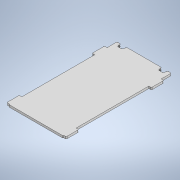
# Autodesk Inventor part: back_wall
Saved by Autodesk Inventor 2020 (Build 240168000, 168)
## iProperties
Created: 2019-06-12
Part Number: back_wall
Material: Generic
Document SubType Name: Modeling
Designer: Dammy
Density: 1 g/cm^3
Appearance: Default
Author: Dammy
Autodesk Inventor part; units mm, degrees
ref_plane "YZ Plane" through (0, 0, 0) normal (1, 0, 0) x (0, 1, 0)
ref_plane "XZ Plane" through (0, 0, 0) normal (0, 1, 0) x (-1, 0, 0)
ref_plane "XY Plane" through (0, 0, 0) normal (0, 0, 1) x (1, 0, 0)
sketch "Sketch1" plane through (0, 0, 0) normal (0, 1, 0) x (-1, 0, 0)
  line L0 (-2, -229.675) -> (-6, -229.675)
  line L1 (-6, -200.675) -> (-2, -200.675)
  line L2 (0, -202.675) -> (0, -227.675)
  line L3 (-6, -30.675) -> (-2, -30.675)
  line L4 (0, -28.675) -> (0, -3.675)
  line L5 (-2, -1.675) -> (-6, -1.675)
  arc A0 (0, -3.675) -> (-2, -1.675) centre (-2, -3.675) ccw
  arc A1 (-2, -30.675) -> (0, -28.675) centre (-2, -28.675) ccw
  arc A2 (0, -202.675) -> (-2, -200.675) centre (-2, -202.675) ccw
  arc A3 (-2, -229.675) -> (0, -227.675) centre (-2, -227.675) ccw
  line L6 (-136.5, -229.675) -> (-132.5, -229.675)
  line L7 (-132.5, -200.675) -> (-136.5, -200.675)
  line L8 (-138.5, -202.675) -> (-138.5, -227.675)
  line L9 (-136.5, -30.675) -> (-132.5, -30.675)
  line L10 (-132.5, -1.675) -> (-136.5, -1.675)
  line L11 (-138.5, -3.675) -> (-138.5, -28.675)
  arc A4 (-136.5, -1.675) -> (-138.5, -3.675) centre (-136.5, -3.675) ccw
  arc A5 (-138.5, -28.675) -> (-136.5, -30.675) centre (-136.5, -28.675) ccw
  arc A6 (-136.5, -200.675) -> (-138.5, -202.675) centre (-136.5, -202.675) ccw
  arc A7 (-138.5, -227.675) -> (-136.5, -229.675) centre (-136.5, -227.675) ccw
  line L12 (-27.75, -250) -> (-27.75, -247)
  line L13 (-110.75, -250) -> (-110.75, -247)
  line L14 (-30.75, -253) -> (-107.75, -253)
  line L15 (0, -215.175) -> (-138.5, -215.175) construction
  line L16 (-113.75, -244) -> (-120.45, -244)
  line L17 (-123.45, -247) -> (-123.45, -250)
  line L18 (-126.45, -253) -> (-127.7679, -253)
  line L19 (-24.75, -244) -> (-18.05, -244)
  line L20 (-15.05, -247) -> (-15.05, -250)
  line L21 (-12.05, -253) -> (-8, -253)
  arc A8 (-15.05, -250) -> (-12.05, -253) centre (-12.05, -250) ccw
  arc A9 (-15.05, -247) -> (-18.05, -244) centre (-18.05, -247) ccw
  arc A10 (-24.75, -244) -> (-27.75, -247) centre (-24.75, -247) ccw
  arc A11 (-30.75, -253) -> (-27.75, -250) centre (-30.75, -250) ccw
  arc A12 (-110.75, -250) -> (-107.75, -253) centre (-107.75, -250) ccw
  arc A13 (-110.75, -247) -> (-113.75, -244) centre (-113.75, -247) ccw
  arc A14 (-120.45, -244) -> (-123.45, -247) centre (-120.45, -247) ccw
  arc A15 (-126.45, -253) -> (-123.45, -250) centre (-126.45, -250) ccw
  line L22 (-7.5, 0) -> (-128.9984, 0)
  line L23 (-6, -229.675) -> (-6, -251)
  line L24 (-6, -30.675) -> (-6, -200.675)
  line L25 (-132.5, -30.675) -> (-132.5, -200.675)
  line L26 (-132.5, -229.675) -> (-132.5, -91)
  line L27 (-128.9984, 0) -> (-131.5, 0)
  line L28 (-132.5, -1) -> (-132.5, -1.675)
  arc A16 (-131.5, 0) -> (-132.5, -1) centre (-131.5, -1) ccw
  line L29 (-6, -1.675) -> (-6, -1)
  line L30 (-6, 0) -> (-6, 0)
  line L31 (-7, 0) -> (-7.5, 0)
  arc A17 (-6, -1) -> (-7, 0) centre (-7, -1) ccw
  line L32 (-132.5, -91) -> (-132.5, -251)
  line L33 (-130.5, -253) -> (-127.109, -253)
  arc A18 (-132.5, -251) -> (-130.5, -253) centre (-130.5, -251) ccw
  line L34 (-4.5, -253) -> (-10.025, -253)
  arc A19 (-8, -253) -> (-6, -251) centre (-8, -251) ccw
  point P0 (0, 0)
  point P1 (0, -229.675)
  point P2 (-4, -229.675)
  point P3 (-138.5, -200.675)
  point P4 (-138.5, -30.675)
  point P5 (-134.5, -229.675)
  point P6 (-132.5, -253)
  point P7 (-27.75, -253)
  point P8 (-27.75, -244)
  point P9 (-110.75, -253)
  point P10 (-110.75, -244)
  point P11 (-69.25, -253)
  point P12 (-69.25, -215.175)
  point P13 (-123.45, -244)
  point P14 (-15.05, -244)
  point P15 (-6.4873, -253)
  point P16 (-6, -91.775)
  point P17 (-4, -1.675)
  point P18 (-134.5, -1.675)
  point P19 (0, -16.175)
  point P20 (-6, -240.3375)
  point P21 (-6, -115.675)
  point P22 (-132.5, -160.3375)
  point P23 (-132.5, -115.675)
  point P24 (-138.5, -16.175)
  point P25 (-132.5, -1.3375)
  point P26 (-134.5, -30.675)
  point P27 (-4, -30.675)
  point P28 (-4, -200.675)
  point P29 (-134.5, -200.675)
  dimension "d3" = 6
  dimension "d8" = 2
  dimension "d11" = 2
  dimension "d12" = 2
  dimension "d13" = 9
  dimension "d14" = 83
  dimension "d15" = 12.7
  dimension "d16" = 12.7
  dimension "d18" = 3
  dimension "d19" = 3
  dimension "d24" = 6
  dimension "d25" = 1
  dimension "d26" = 1
  dimension "d29" = 29
  dimension "d30" = 23.325
  dimension "d31" = 2
  dimension "d34" = 2
  dimension "d35" = 126.5
  dimension "d36" = 244
  dimension "d37" = 29
  dimension "d38" = 1.675
  constraints: 70 end point, 40 point on circle, 40 tangent, 28 point on line, 21 midpoint, 20 centre point, 13 vertical alignment, 11 equal radius, 11 horizontal alignment, 9 horizontal, 6 parallel, 6 perpendicular, 6 vertical, 3 collinear
  measures "d3" distance of point (0, -229.675) L0.end
  measures "d8" radius of A0
  measures "d11" radius of A4
  measures "d12" radius of A6
  measures "d13" distance of point (-27.75, -253) point (-27.75, -244)
  measures "d14" distance between parallel lines of L13 L12
  measures "d15" distance of point (-110.75, -244) point (-123.45, -244)
  measures "d16" distance of point (-27.75, -244) point (-15.05, -244)
  measures "d18" radius of A8
  measures "d19" radius of A12
  measures "d24" distance between parallel lines of L8 L26
  measures "d25" radius of A16
  measures "d26" radius of A17
  measures "d29" distance from line of L1 point (-4, -229.675)
  measures "d30" distance from line of L21 point (-4, -229.675)
  measures "d31" radius of A18
  measures "d34" radius of A19
  measures "d35" distance between parallel lines of L26 L23
  measures "d36" distance between parallel lines of L22 L16
  measures "d37" vertical distance of L3.end point (-4, -1.675)
  measures "d38" distance from line of L22 L5.start
extrude "Extrusion1" add sketch "Sketch1" along normal blind 5
equation "\"d19\" = d18"
equation "\"d24\" = d3"
equation "\"d25\" = d26"
equation "\"d31\" = d17"
equation "\"d37\" = d29"
equation "\"d17\" = 2"
body "Solid1"
